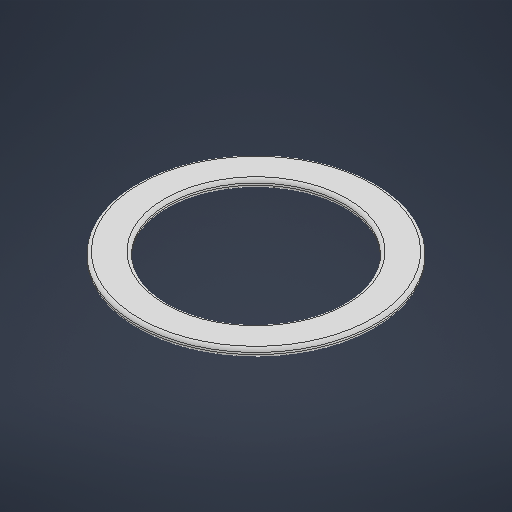
# Autodesk Inventor part: Coil
Saved by Autodesk Inventor 2026.1 (Build 301233020, 233B)
## iProperties
Created: 2026-05-23
Part Number: Coil
Material: Generic
Document SubType Name: Modeling
Designer: InventorKid
Density: 1 g/cm^3
Appearance: Default
Author: InventorKid
Autodesk Inventor part; units mm, degrees
ref_plane "YZ Plane" through (0, 0, 0) normal (1, 0, 0) x (0, 1, 0)
ref_plane "XZ Plane" through (0, 0, 0) normal (0, 1, 0) x (-1, 0, 0)
ref_plane "XY Plane" through (0, 0, 0) normal (0, 0, 1) x (1, 0, 0)
sketch "Sketch1" plane through (0, 0, 0) normal (0, 1, 0) x (-1, 0, 0)
  circle A0 centre (0, 0) radius 14
  circle A1 centre (0, 0) radius 19
  dimension "d0" = 28
  dimension "d1" = 38
  constraints: 2 centre point, 2 coincident
  measures "d0" diameter of A0
  measures "d1" diameter of A1
extrude "Extrusion1" add sketch "Sketch1" along normal blind 1.3
fillet "Fillet1" radius 0.5 4 edges at (19, 1.3, 0) (19, 0, 0) (14, 1.3, 0) (14, 0, 0)
body "Solid1"
